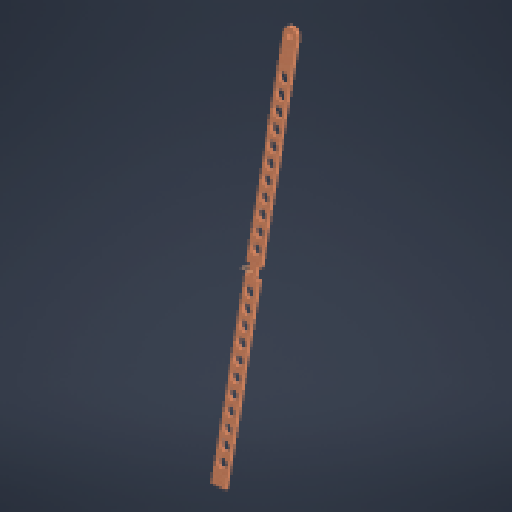
# Autodesk Inventor part: UPRIGHTS_TREBUCHET
Saved by Autodesk Inventor 2026.2 (Build 302298010, 298A)
## iProperties
Created: 2026-02-18
Part Number: UPRIGHTS_TREBUCHET
Material: Wood (Oak)
Document SubType Name: Modeling
Designer: 4aida
Density: 0.76 g/cm^3
Appearance: White Oak - Natural Medium Gloss
Mass: 194.688 g
Surface Area: 913.544 cm^2
Volume: 256.168 cm^3
Author: 4aida
Autodesk Inventor part; units mm, degrees
ref_plane "YZ Plane" through (0, 0, 0) normal (1, 0, 0) x (0, 1, 0)
ref_plane "XZ Plane" through (0, 0, 0) normal (0, 1, 0) x (-1, 0, 0)
ref_plane "XY Plane" through (0, 0, 0) normal (0, 0, 1) x (1, 0, 0)
sketch "Sketch1" plane through (0, 0, 0) normal (1, 0, 0) x (0, 1, 0)
  line L0 (0, 4.8581) -> (0, -4.8581)
  line L1 (0, 4.8581) -> (1000, -196.5631)
  line L2 (1000, -196.5631) -> (1000, -206.2794)
  line L3 (1000, -206.2794) -> (0, -4.8581)
  point P0 (0, 0)
  point P1 (0, 0)
  dimension "d0" = 9.525
  dimension "d1" = 1000
  dimension "d9" = 211.1375
  dimension "d10" = 78.612
  constraints: 8 end point, 2 parallel, 1 coincident, 1 midpoint, 1 vertical
  measures "d0" distance between parallel lines of L3 L1
  measures "d1" distance between parallel lines of L0 L2
  measures "d9" vertical distance of L2.end L0.start
  measures "d10" angle of L3 L0
extrude "Extrusion1" add sketch "Sketch1" along normal mid plane 38.1
sketch "Sketch2" plane through (0, 0, 0) normal (0, 0, 1) x (1, 0, 0)
  circle A0 centre (0, 980.95) radius 6.35
  circle A1 centre (0, 980.95) radius 19.05
  line L0 (19.05, 1000) -> (19.05, 0) projected
  line L1 (-19.05, 1000) -> (19.05, 1000) projected
  line L2 (-19.05, 1000) -> (-19.05, 980.95)
  point P0 (0, 0)
  point P1 (0, 1000)
  point P2 (19.05, 980.95)
  dimension "d5" = 38.1
  dimension "d6" = 12.7
  constraints: 2 end point, 2 vertical, 1 centre point, 1 coincident, 1 horizontal, 3 other
  measures "d6" diameter of A0
extrude "Extrusion2" cut sketch "Sketch2" along normal through all both and the other way through all contours A0 | L2 L1 A1 | A1 L1 L0
sketch "Sketch3" plane through (-19.05, 0, 4.8581) normal (0, 0.1974556, 0.9803118) x (1, 0, 0)
  line L0 (0, 1002.5695) -> (0, 1.9185) projected
  line L1 (0, 493.095) -> (9.525, 495)
  line L2 (9.525, 495) -> (9.525, 465)
  line L3 (9.525, 465) -> (0, 466.905)
  line L4 (38.1, 0) -> (0, 0) projected
  line L5 (0, 493.095) -> (9.525, 493.095) construction
  point P0 (19.05, 0.9593)
  point P1 (9.525, 480)
  dimension "d11" = 9.525
  dimension "d12" = 480
  dimension "d14" = 1.905
  dimension "d15" = 30
  constraints: 8 end point, 2 point on line, 1 equal length, 1 horizontal, 1 midpoint, 1 parallel
  measures "d11" distance between parallel lines of L2 L0
  measures "d12" distance from line of L4 point (9.525, 480)
  measures "d14" distance from line of L1.end L5
  measures "d15" distance of L1.end L2.end
extrude "Extrusion3" cut sketch "Sketch3" against normal blind 10
mirror "Mirror1" about plane through (0, 0, 0) normal (1, 0, 0) of "Extrusion3"
sketch "Sketch4" plane through (-19.05, 0, 4.8581) normal (0, 0.1974556, 0.9803118) x (1, 0, 0)
  circle A0 centre (19.05, 51.7593) radius 12.7
  line L0 (38.1, 466.905) -> (38.1, 0) projected
  circle A1 centre (19.05, 89.8593) radius 12.7
  circle A2 centre (19.05, 127.9593) radius 12.7
  circle A3 centre (19.05, 166.0593) radius 12.7
  circle A4 centre (19.05, 204.1593) radius 12.7
  circle A5 centre (19.05, 242.2593) radius 12.7
  circle A6 centre (19.05, 280.3593) radius 12.7
  circle A7 centre (19.05, 318.4593) radius 12.7
  circle A8 centre (19.05, 356.5593) radius 12.7
  circle A9 centre (19.05, 394.6593) radius 12.7
  circle A10 centre (19.05, 432.7593) radius 12.7
  point P0 (19.05, 0.9593)
  dimension "d18" = 25.4
  dimension "d19" = 50.8
  dimension "d22" = 38.1
  constraints: 11 centre point, 1 vertical, 1 vertical alignment, 20 other
  measures "d18" diameter of A0
  measures "d19" distance of point (19.05, 0.959) A0.centre
  measures "d22" distance of A0.centre A1.centre
extrude "Extrusion4" cut sketch "Sketch4" against normal through all
ref_plane "Work Plane1" through (-9.525, 470.5497, -89.9205) normal (0, 0.9803118, -0.1974556) x (-1, 0, 0)
mirror "Mirror2" about plane through (-9.525, 470.5497, -89.9205) normal (0, 0.9803118, -0.1974556) of "Extrusion4"
equation "\"d14\" = 0.2 * d11"
body "Solid1"
